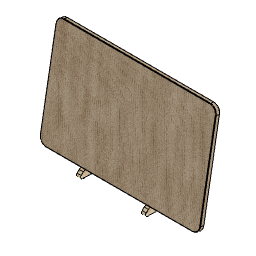
model (Autodesk Fusion 360 design; units mm, degrees)
Autodesk Fusion 360 part; units mm, degrees
note: some values were not read from the file. Chosen so that the rebuilt part matches the saved one: which bodies a step acts on; which face or edge a step refers to.
sketch "Sketch1" plane through (0, 0, 0) normal (0, 0, 1) x (1, 0, 0) in component "stock"
  line L0 (0, 0) -> (184.15, 0)
  line L1 (184.15, 0) -> (184.15, 1168.4)
  line L2 (184.15, 1168.4) -> (0, 1168.4)
  line L3 (0, 1168.4) -> (0, 0)
  line L4 (-207.15, 0) -> (-23, 0)
  line L5 (-23, 0) -> (-23, 28)
  line L6 (-23, 28) -> (-207.15, 28)
  line L7 (-207.15, 28) -> (-207.15, 0)
  line L8 (-207.15, 30) -> (-23, 30)
  line L9 (-23, 30) -> (-23, 58)
  line L10 (-207.15, 58) -> (-207.15, 30)
  line L11 (-23, 58) -> (-207.15, 58)
  line L12 (-207.15, 60) -> (-23, 60)
  line L13 (-23, 60) -> (-23, 88)
  line L14 (-207.15, 88) -> (-207.15, 60)
  line L15 (-23, 88) -> (-207.15, 88)
  line L16 (-207.15, 90) -> (-23, 90)
  line L17 (-23, 90) -> (-23, 118)
  line L18 (-207.15, 118) -> (-207.15, 90)
  line L19 (-23, 118) -> (-207.15, 118)
  line L20 (-207.15, 120) -> (-23, 120)
  line L21 (-23, 120) -> (-23, 148)
  line L22 (-207.15, 148) -> (-207.15, 120)
  line L23 (-23, 148) -> (-207.15, 148)
  line L24 (-207.15, 150) -> (-23, 150)
  line L25 (-23, 150) -> (-23, 178)
  line L26 (-207.15, 178) -> (-207.15, 150)
  line L27 (-23, 178) -> (-207.15, 178)
  line L28 (-207.15, 180) -> (-23, 180)
  line L29 (-23, 180) -> (-23, 208)
  line L30 (-207.15, 208) -> (-207.15, 180)
  line L31 (-23, 208) -> (-207.15, 208)
  line L32 (-207.15, 210) -> (-23, 210)
  line L33 (-23, 210) -> (-23, 238)
  line L34 (-207.15, 238) -> (-207.15, 210)
  line L35 (-23, 238) -> (-207.15, 238)
  line L36 (-207.15, 240) -> (-23, 240)
  line L37 (-23, 240) -> (-23, 268)
  line L38 (-207.15, 268) -> (-207.15, 240)
  line L39 (-23, 268) -> (-207.15, 268)
  line L40 (-207.15, 270) -> (-23, 270)
  line L41 (-23, 270) -> (-23, 298)
  line L42 (-207.15, 298) -> (-207.15, 270)
  line L43 (-23, 298) -> (-207.15, 298)
  line L44 (-207.15, 300) -> (-23, 300)
  line L45 (-23, 300) -> (-23, 328)
  line L46 (-207.15, 328) -> (-207.15, 300)
  line L47 (-23, 328) -> (-207.15, 328)
  line L48 (-207.15, 330) -> (-23, 330)
  line L49 (-23, 330) -> (-23, 358)
  line L50 (-207.15, 358) -> (-207.15, 330)
  line L51 (-23, 358) -> (-207.15, 358)
  line L52 (-207.15, 360) -> (-23, 360)
  line L53 (-23, 360) -> (-23, 388)
  line L54 (-207.15, 388) -> (-207.15, 360)
  line L55 (-23, 388) -> (-207.15, 388)
  line L56 (-207.15, 390) -> (-23, 390)
  line L57 (-23, 390) -> (-23, 418)
  line L58 (-207.15, 418) -> (-207.15, 390)
  line L59 (-23, 418) -> (-207.15, 418)
  line L60 (-207.15, 420) -> (-23, 420)
  line L61 (-23, 420) -> (-23, 448)
  line L62 (-207.15, 448) -> (-207.15, 420)
  line L63 (-23, 448) -> (-207.15, 448)
  line L64 (-207.15, 450) -> (-23, 450)
  line L65 (-23, 450) -> (-23, 478)
  line L66 (-207.15, 478) -> (-207.15, 450)
  line L67 (-23, 478) -> (-207.15, 478)
  line L68 (-207.15, 480) -> (-23, 480)
  line L69 (-23, 480) -> (-23, 508)
  line L70 (-207.15, 508) -> (-207.15, 480)
  line L71 (-23, 508) -> (-207.15, 508)
  line L72 (-207.15, 510) -> (-23, 510)
  line L73 (-23, 510) -> (-23, 538)
  line L74 (-207.15, 538) -> (-207.15, 510)
  line L75 (-23, 538) -> (-207.15, 538)
  line L76 (-207.15, 540) -> (-23, 540)
  line L77 (-23, 540) -> (-23, 568)
  line L78 (-207.15, 568) -> (-207.15, 540)
  line L79 (-23, 568) -> (-207.15, 568)
  line L80 (-207.15, 570) -> (-23, 570)
  line L81 (-23, 570) -> (-23, 598)
  line L82 (-207.15, 598) -> (-207.15, 570)
  line L83 (-23, 598) -> (-207.15, 598)
  line L84 (-207.15, 600) -> (-23, 600)
  line L85 (-23, 600) -> (-23, 628)
  line L86 (-207.15, 628) -> (-207.15, 600)
  line L87 (-23, 628) -> (-207.15, 628)
  line L88 (-207.15, 630) -> (-23, 630)
  line L89 (-23, 630) -> (-23, 658)
  line L90 (-207.15, 658) -> (-207.15, 630)
  line L91 (-23, 658) -> (-207.15, 658)
  line L92 (-207.15, 660) -> (-23, 660)
  line L93 (-23, 660) -> (-23, 688)
  line L94 (-207.15, 688) -> (-207.15, 660)
  line L95 (-23, 688) -> (-207.15, 688)
  line L96 (-207.15, 690) -> (-23, 690)
  line L97 (-23, 690) -> (-23, 718)
  line L98 (-207.15, 718) -> (-207.15, 690)
  line L99 (-23, 718) -> (-207.15, 718)
  line L100 (-207.15, 720) -> (-23, 720)
  line L101 (-23, 720) -> (-23, 748)
  line L102 (-207.15, 748) -> (-207.15, 720)
  line L103 (-23, 748) -> (-207.15, 748)
  line L104 (-207.15, 750) -> (-23, 750)
  line L105 (-23, 750) -> (-23, 778)
  line L106 (-207.15, 778) -> (-207.15, 750)
  line L107 (-23, 778) -> (-207.15, 778)
  line L108 (-207.15, 780) -> (-23, 780)
  line L109 (-23, 780) -> (-23, 808)
  line L110 (-207.15, 808) -> (-207.15, 780)
  line L111 (-23, 808) -> (-207.15, 808)
  line L112 (-207.15, 810) -> (-23, 810)
  line L113 (-23, 810) -> (-23, 838)
  line L114 (-207.15, 838) -> (-207.15, 810)
  line L115 (-23, 838) -> (-207.15, 838)
  line L116 (-207.15, 840) -> (-23, 840)
  line L117 (-23, 840) -> (-23, 868)
  line L118 (-207.15, 868) -> (-207.15, 840)
  line L119 (-23, 868) -> (-207.15, 868)
  line L120 (-207.15, 870) -> (-23, 870)
  line L121 (-23, 870) -> (-23, 898)
  line L122 (-207.15, 898) -> (-207.15, 870)
  line L123 (-23, 898) -> (-207.15, 898)
  line L124 (-207.15, 900) -> (-23, 900)
  line L125 (-23, 900) -> (-23, 928)
  line L126 (-207.15, 928) -> (-207.15, 900)
  line L127 (-23, 928) -> (-207.15, 928)
  line L128 (-207.15, 930) -> (-23, 930)
  line L129 (-23, 930) -> (-23, 958)
  line L130 (-207.15, 958) -> (-207.15, 930)
  line L131 (-23, 958) -> (-207.15, 958)
  line L132 (-207.15, 960) -> (-23, 960)
  line L133 (-23, 960) -> (-23, 988)
  line L134 (-207.15, 988) -> (-207.15, 960)
  line L135 (-23, 988) -> (-207.15, 988)
  line L136 (207.15, 1168.4) -> (207.15, 0)
  line L137 (207.15, 0) -> (391.3, 0)
  line L138 (391.3, 1168.4) -> (207.15, 1168.4)
  line L139 (391.3, 0) -> (391.3, 1168.4)
  line L140 (414.3, 1168.4) -> (414.3, 0)
  line L141 (414.3, 0) -> (598.45, 0)
  line L142 (598.45, 1168.4) -> (414.3, 1168.4)
  line L143 (598.45, 0) -> (598.45, 1168.4)
  line L144 (-207.15, 990) -> (-23, 990)
  line L145 (-23, 990) -> (-23, 1018)
  line L146 (-207.15, 1018) -> (-207.15, 990)
  line L147 (-23, 1018) -> (-207.15, 1018)
  dimension "d4" = 184.15
  dimension "d5" = 1168.4
  dimension "d19" = 184.15
  dimension "d20" = 28
  dimension "d25" = 0
  dimension "d26" = 30
  dimension "d27" = 23
  dimension "d30" = 207.15
  dimension "d31" = 0
  constraint horizontal L0
  constraint vertical L1
  constraint horizontal L2
  constraint vertical L3
  constraint coincident L0.start L3.end
  constraint horizontal L4
  constraint vertical L5
  constraint horizontal L6
  constraint vertical L7
  constraint collinear L0 L4
  measures "d4" distance of L1.end L2.end
  measures "d5" distance of L0.start L2.end
  measures "d19" distance of L4.start L4.end
  measures "d20" distance of L4.start L6.end
  measures "d27" distance of L3 L5
sketch "Sketch1 (2)" plane through (0, 0, 0) normal (0, 0, 1) x (1, 0, 0) in component "layout"
  line L0 (-795, -650) -> (-100, -650)
  line L1 (-100, -650) -> (-100, -200)
  line L2 (-100, -200) -> (-795, -200)
  line L3 (-795, -200) -> (-795, -650)
  line L4 (100, -200) -> (146.5, -200)
  line L5 (146.5, -200) -> (146.5, -384.15)
  line L6 (146.5, -384.15) -> (100, -384.15)
  line L7 (100, -384.15) -> (100, -200)
  line L8 (100, -200) -> (795, -200) construction
  line L9 (795, -200) -> (795, -650) construction
  line L10 (795, -650) -> (100, -650) construction
  line L11 (100, -650) -> (100, -200) construction
  line L12 (193, -384.15) -> (193, -200)
  line L13 (193, -200) -> (239.5, -200)
  line L14 (239.5, -384.15) -> (193, -384.15)
  line L15 (239.5, -200) -> (239.5, -384.15)
  line L16 (286, -384.15) -> (286, -200)
  line L17 (286, -200) -> (332.5, -200)
  line L18 (332.5, -384.15) -> (286, -384.15)
  line L19 (332.5, -200) -> (332.5, -384.15)
  line L20 (379, -384.15) -> (379, -200)
  line L21 (379, -200) -> (425.5, -200)
  line L22 (425.5, -384.15) -> (379, -384.15)
  line L23 (425.5, -200) -> (425.5, -384.15)
  line L24 (100, -568.3) -> (100, -384.15)
  line L25 (100, -384.15) -> (146.5, -384.15)
  line L26 (146.5, -568.3) -> (100, -568.3)
  line L27 (146.5, -384.15) -> (146.5, -568.3)
  line L28 (193, -568.3) -> (193, -384.15)
  line L29 (193, -384.15) -> (239.5, -384.15)
  line L30 (239.5, -568.3) -> (193, -568.3)
  line L31 (239.5, -384.15) -> (239.5, -568.3)
  line L32 (286, -568.3) -> (286, -384.15)
  line L33 (286, -384.15) -> (332.5, -384.15)
  line L34 (332.5, -568.3) -> (286, -568.3)
  line L35 (332.5, -384.15) -> (332.5, -568.3)
  line L36 (379, -568.3) -> (379, -384.15)
  line L37 (379, -384.15) -> (425.5, -384.15)
  line L38 (425.5, -568.3) -> (379, -568.3)
  line L39 (425.5, -384.15) -> (425.5, -568.3)
  line L40 (100, -752.45) -> (100, -568.3)
  line L41 (100, -568.3) -> (146.5, -568.3)
  line L42 (146.5, -752.45) -> (100, -752.45)
  line L43 (146.5, -568.3) -> (146.5, -752.45)
  line L44 (193, -752.45) -> (193, -568.3)
  line L45 (193, -568.3) -> (239.5, -568.3)
  line L46 (239.5, -752.45) -> (193, -752.45)
  line L47 (239.5, -568.3) -> (239.5, -752.45)
  line L48 (286, -752.45) -> (286, -568.3)
  line L49 (286, -568.3) -> (332.5, -568.3)
  line L50 (332.5, -752.45) -> (286, -752.45)
  line L51 (332.5, -568.3) -> (332.5, -752.45)
  line L52 (379, -752.45) -> (379, -568.3)
  line L53 (379, -568.3) -> (425.5, -568.3)
  line L54 (425.5, -752.45) -> (379, -752.45)
  line L55 (425.5, -568.3) -> (425.5, -752.45)
  line L56 (-744.2, -599.2) -> (-150.8, -599.2) construction
  line L57 (-150.8, -599.2) -> (-150.8, -250.8) construction
  line L58 (-150.8, -250.8) -> (-744.2, -250.8) construction
  line L59 (-744.2, -250.8) -> (-744.2, -599.2) construction
  circle A0 centre (-744.2, -250.8) radius 9.525
  circle A1 centre (-150.8, -250.8) radius 9.525
  circle A2 centre (-150.8, -599.2) radius 9.525
  circle A3 centre (-744.2, -599.2) radius 9.525
  line L60 (472, -384.15) -> (472, -200)
  line L61 (472, -200) -> (518.5, -200)
  line L62 (518.5, -384.15) -> (472, -384.15)
  line L63 (518.5, -200) -> (518.5, -384.15)
  line L64 (565, -384.15) -> (565, -200)
  line L65 (565, -200) -> (611.5, -200)
  line L66 (611.5, -384.15) -> (565, -384.15)
  line L67 (611.5, -200) -> (611.5, -384.15)
  line L68 (658, -384.15) -> (658, -200)
  line L69 (658, -200) -> (704.5, -200)
  line L70 (704.5, -384.15) -> (658, -384.15)
  line L71 (704.5, -200) -> (704.5, -384.15)
  line L72 (751, -384.15) -> (751, -200)
  line L73 (751, -200) -> (797.5, -200)
  line L74 (797.5, -384.15) -> (751, -384.15)
  line L75 (797.5, -200) -> (797.5, -384.15)
  line L76 (472, -568.3) -> (472, -384.15)
  line L77 (472, -384.15) -> (518.5, -384.15)
  line L78 (518.5, -568.3) -> (472, -568.3)
  line L79 (518.5, -384.15) -> (518.5, -568.3)
  line L80 (565, -568.3) -> (565, -384.15)
  line L81 (565, -384.15) -> (611.5, -384.15)
  line L82 (611.5, -568.3) -> (565, -568.3)
  line L83 (611.5, -384.15) -> (611.5, -568.3)
  line L84 (658, -568.3) -> (658, -384.15)
  line L85 (658, -384.15) -> (704.5, -384.15)
  line L86 (704.5, -568.3) -> (658, -568.3)
  line L87 (704.5, -384.15) -> (704.5, -568.3)
  line L88 (751, -568.3) -> (751, -384.15)
  line L89 (751, -384.15) -> (797.5, -384.15)
  line L90 (797.5, -568.3) -> (751, -568.3)
  line L91 (797.5, -384.15) -> (797.5, -568.3)
  line L92 (472, -752.45) -> (472, -568.3)
  line L93 (472, -568.3) -> (518.5, -568.3)
  line L94 (518.5, -752.45) -> (472, -752.45)
  line L95 (518.5, -568.3) -> (518.5, -752.45)
  line L96 (565, -752.45) -> (565, -568.3)
  line L97 (565, -568.3) -> (611.5, -568.3)
  line L98 (611.5, -752.45) -> (565, -752.45)
  line L99 (611.5, -568.3) -> (611.5, -752.45)
  line L100 (658, -752.45) -> (658, -568.3)
  line L101 (658, -568.3) -> (704.5, -568.3)
  line L102 (704.5, -752.45) -> (658, -752.45)
  line L103 (704.5, -568.3) -> (704.5, -752.45)
  line L104 (751, -752.45) -> (751, -568.3)
  line L105 (751, -568.3) -> (797.5, -568.3)
  line L106 (797.5, -752.45) -> (751, -752.45)
  line L107 (797.5, -568.3) -> (797.5, -752.45)
  line L108 (146.5, -292.075) -> (193, -292.075)
  line L109 (193, -292.075) -> (193, -107.925)
  line L110 (193, -107.925) -> (146.5, -107.925)
  line L111 (146.5, -107.925) -> (146.5, -292.075)
  line L112 (286, -292.075) -> (286, -107.925)
  line L113 (286, -107.925) -> (239.5, -107.925)
  line L114 (239.5, -107.925) -> (239.5, -292.075)
  line L115 (239.5, -292.075) -> (286, -292.075)
  line L116 (379, -292.075) -> (379, -107.925)
  line L117 (379, -107.925) -> (332.5, -107.925)
  line L118 (332.5, -107.925) -> (332.5, -292.075)
  line L119 (332.5, -292.075) -> (379, -292.075)
  line L120 (472, -292.075) -> (472, -107.925)
  line L121 (472, -107.925) -> (425.5, -107.925)
  line L122 (425.5, -107.925) -> (425.5, -292.075)
  line L123 (425.5, -292.075) -> (472, -292.075)
  line L124 (565, -292.075) -> (565, -107.925)
  line L125 (565, -107.925) -> (518.5, -107.925)
  line L126 (518.5, -107.925) -> (518.5, -292.075)
  line L127 (518.5, -292.075) -> (565, -292.075)
  line L128 (658, -292.075) -> (658, -107.925)
  line L129 (658, -107.925) -> (611.5, -107.925)
  line L130 (611.5, -107.925) -> (611.5, -292.075)
  line L131 (611.5, -292.075) -> (658, -292.075)
  line L132 (751, -292.075) -> (751, -107.925)
  line L133 (751, -107.925) -> (704.5, -107.925)
  line L134 (704.5, -107.925) -> (704.5, -292.075)
  line L135 (704.5, -292.075) -> (751, -292.075)
  line L136 (193, -476.225) -> (193, -292.075)
  line L137 (193, -292.075) -> (146.5, -292.075)
  line L138 (146.5, -292.075) -> (146.5, -476.225)
  line L139 (146.5, -476.225) -> (193, -476.225)
  line L140 (286, -476.225) -> (286, -292.075)
  line L141 (286, -292.075) -> (239.5, -292.075)
  line L142 (239.5, -292.075) -> (239.5, -476.225)
  line L143 (239.5, -476.225) -> (286, -476.225)
  line L144 (379, -476.225) -> (379, -292.075)
  line L145 (379, -292.075) -> (332.5, -292.075)
  line L146 (332.5, -292.075) -> (332.5, -476.225)
  line L147 (332.5, -476.225) -> (379, -476.225)
  line L148 (472, -476.225) -> (472, -292.075)
  line L149 (472, -292.075) -> (425.5, -292.075)
  line L150 (425.5, -292.075) -> (425.5, -476.225)
  line L151 (425.5, -476.225) -> (472, -476.225)
  line L152 (565, -476.225) -> (565, -292.075)
  line L153 (565, -292.075) -> (518.5, -292.075)
  line L154 (518.5, -292.075) -> (518.5, -476.225)
  line L155 (518.5, -476.225) -> (565, -476.225)
  line L156 (658, -476.225) -> (658, -292.075)
  line L157 (658, -292.075) -> (611.5, -292.075)
  line L158 (611.5, -292.075) -> (611.5, -476.225)
  line L159 (611.5, -476.225) -> (658, -476.225)
  line L160 (751, -476.225) -> (751, -292.075)
  line L161 (751, -292.075) -> (704.5, -292.075)
  line L162 (704.5, -292.075) -> (704.5, -476.225)
  line L163 (704.5, -476.225) -> (751, -476.225)
  line L164 (193, -660.375) -> (193, -476.225)
  line L165 (193, -476.225) -> (146.5, -476.225)
  line L166 (146.5, -476.225) -> (146.5, -660.375)
  line L167 (146.5, -660.375) -> (193, -660.375)
  line L168 (286, -660.375) -> (286, -476.225)
  line L169 (286, -476.225) -> (239.5, -476.225)
  line L170 (239.5, -476.225) -> (239.5, -660.375)
  line L171 (239.5, -660.375) -> (286, -660.375)
  line L172 (379, -660.375) -> (379, -476.225)
  line L173 (379, -476.225) -> (332.5, -476.225)
  line L174 (332.5, -476.225) -> (332.5, -660.375)
  line L175 (332.5, -660.375) -> (379, -660.375)
  line L176 (472, -660.375) -> (472, -476.225)
  line L177 (472, -476.225) -> (425.5, -476.225)
  line L178 (425.5, -476.225) -> (425.5, -660.375)
  line L179 (425.5, -660.375) -> (472, -660.375)
  line L180 (565, -660.375) -> (565, -476.225)
  line L181 (565, -476.225) -> (518.5, -476.225)
  line L182 (518.5, -476.225) -> (518.5, -660.375)
  line L183 (518.5, -660.375) -> (565, -660.375)
  line L184 (658, -660.375) -> (658, -476.225)
  line L185 (658, -476.225) -> (611.5, -476.225)
  line L186 (611.5, -476.225) -> (611.5, -660.375)
  line L187 (611.5, -660.375) -> (658, -660.375)
  line L188 (751, -660.375) -> (751, -476.225)
  line L189 (751, -476.225) -> (704.5, -476.225)
  line L190 (704.5, -476.225) -> (704.5, -660.375)
  line L191 (704.5, -660.375) -> (751, -660.375)
  dimension "d14" = 695
  dimension "d15" = 450
  dimension "d36" = 200
  dimension "d38" = 100
  dimension "d39" = 46.5
  dimension "d40" = 184.15
  dimension "d41" = 200
  dimension "d42" = 695
  dimension "d43" = 450
  dimension "d46" = 93
  dimension "d79" = 19.05
  dimension "d80" = 19.05
  dimension "d81" = 19.05
  dimension "d82" = 19.05
  dimension "d98" = 93
  constraint horizontal L0
  constraint vertical L1
  constraint horizontal L2
  constraint vertical L3
  constraint horizontal L4
  constraint vertical L5
  constraint horizontal L6
  constraint vertical L7
  constraint collinear L2 L4
  constraint horizontal L8
  constraint vertical L9
  constraint horizontal L10
  constraint vertical L11
  constraint coincident L58.end L59.start
  constraint coincident L57.end L58.start
  constraint coincident L56.end L57.start
  constraint coincident L56.start L59.end
  constraint horizontal L108
  constraint vertical L109
  constraint horizontal L110
  constraint vertical L111
  constraint midpoint L5 L108.start
  constraint collinear L12 L109
  constraint equal L7 L111
  measures "d14" distance of L1.end L2.end
  measures "d15" distance of L0.start L2.end
  measures "d36" distance of L2 origin
  measures "d38" distance of origin L1
  measures "d39" distance of L4.start L4.end
  measures "d40" distance of L4.start L6.end
  measures "d41" distance of L1 L7
  measures "d42" distance of L4.start L8.end
  measures "d43" distance of L8.end L9.end
  measures "d79" diameter of A0
  measures "d80" diameter of A1
  measures "d81" diameter of A3
  measures "d82" diameter of A2
extrude "Extrude2" add sketch "Sketch1" along normal blind 46.5 contours L0 L1 L2 L3 makes body 1 in component "stock"
extrude "Extrude3" add sketch "Sketch1" along normal blind 46.5 separate body contours L4 L5 L6 L7 makes body 2 in component "stock"
sketch "Sketch2" plane through (0, 0, 0) normal (0, 0, 1) x (1, 0, 0) in component "brick (outdated)"
  line L0 (0, -0.2486) -> (129.54, -0.2486)
  line L1 (129.54, -0.2486) -> (129.54, 46.2514)
  line L2 (129.54, 46.2514) -> (0, 46.2514)
  line L3 (0, 46.2514) -> (0, -0.2486)
  line L4 (129.54, -0.2486) -> (302.26, -0.2486)
  line L5 (302.26, -0.2486) -> (302.26, 46.2514)
  line L6 (302.26, 46.2514) -> (129.54, 46.2514)
  line L7 (129.54, 46.2514) -> (129.54, -0.2486)
  line L8 (302.26, -0.2486) -> (431.8, -0.2486)
  line L9 (431.8, -0.2486) -> (431.8, 46.2514)
  line L10 (431.8, 46.2514) -> (302.26, 46.2514)
  line L11 (302.26, 46.2514) -> (302.26, -0.2486)
  line L12 (431.8, -0.2486) -> (584.2, -0.2486)
  line L13 (584.2, -0.2486) -> (584.2, 46.2514)
  line L14 (584.2, 46.2514) -> (431.8, 46.2514)
  line L15 (431.8, 46.2514) -> (431.8, -0.2486)
  line L16 (584.2, -0.2486) -> (736.6, -0.2486)
  line L17 (736.6, -0.2486) -> (736.6, 46.2514)
  line L18 (736.6, 46.2514) -> (584.2, 46.2514)
  line L19 (584.2, 46.2514) -> (584.2, -0.2486)
  line L20 (736.6, -0.2486) -> (909.32, -0.2486)
  line L21 (909.32, -0.2486) -> (909.32, 46.2514)
  line L22 (909.32, 46.2514) -> (736.6, 46.2514)
  line L23 (736.6, 46.2514) -> (736.6, -0.2486)
  line L24 (606.8221, -46.2418) -> (779.5421, -46.3005)
  line L25 (324.88, 0.0519) -> (172.4798, 0.0264)
  line L26 (606.821, -46.2418) -> (606.8213, 0.101)
  line L27 (477.2805, 0.0783) -> (477.281, -46.1978)
  line L28 (324.88, 0.0519) -> (324.8803, -46.146)
  line L29 (324.8803, -46.146) -> (477.2803, -46.1978)
  line L30 (172.4798, 0.0264) -> (-0.2403, 0)
  line L31 (477.2805, 0.0783) -> (324.88, 0.0519)
  line L32 (-0.2403, 0) -> (-0.2404, -46.0356)
  line L33 (-0.2404, -46.0356) -> (172.4796, -46.0942)
  line L34 (172.4796, -46.0942) -> (172.4798, 0.0264)
  line L35 (172.4798, 0.0264) -> (172.4798, -46.0942)
  line L36 (324.8798, -46.146) -> (324.88, 0.0519)
  line L37 (779.5437, -46.3005) -> (909.0837, -46.3445)
  line L38 (779.5421, -46.3005) -> (779.5425, 0.1322)
  line L39 (477.281, -46.1978) -> (606.821, -46.2418)
  line L40 (909.078, 0.1555) -> (779.5425, 0.1322)
  line L41 (909.0837, -46.3445) -> (909.078, 0.1555)
  line L42 (606.8213, 0.101) -> (477.2805, 0.0783)
  line L43 (779.5425, 0.1322) -> (606.8213, 0.101)
  line L44 (779.5425, 0.1322) -> (779.5437, -46.3005)
  line L45 (606.8213, 0.101) -> (606.8221, -46.2418)
  line L46 (172.4798, -46.0942) -> (324.8798, -46.146)
  line L47 (477.2803, -46.1978) -> (477.2805, 0.0783)
  line L48 (-0.2404, -139.0356) -> (172.4796, -139.0942)
  line L49 (324.88, -92.9481) -> (324.8803, -139.146)
  line L50 (129.54, -46.7486) -> (0, -46.7486)
  line L51 (584.2, -93.2486) -> (736.6, -93.2486)
  line L52 (431.8, -93.2486) -> (584.2, -93.2486)
  line L53 (324.88, -92.9481) -> (172.4798, -92.9736)
  line L54 (477.281, -139.1978) -> (606.821, -139.2418)
  line L55 (584.2, -46.7486) -> (584.2, -93.2486)
  line L56 (606.8213, -92.899) -> (477.2805, -92.9217)
  line L57 (584.2, -93.2486) -> (584.2, -46.7486)
  line L58 (324.8798, -139.146) -> (324.88, -92.9481)
  line L59 (172.4798, -92.9736) -> (172.4798, -139.0942)
  line L60 (302.26, -93.2486) -> (302.26, -46.7486)
  line L61 (736.6, -46.7486) -> (584.2, -46.7486)
  line L62 (736.6, -93.2486) -> (909.32, -93.2486)
  line L63 (606.8213, -92.899) -> (606.8221, -139.2418)
  line L64 (736.6, -93.2486) -> (736.6, -46.7486)
  line L65 (909.32, -93.2486) -> (909.32, -46.7486)
  line L66 (909.0837, -139.3445) -> (909.078, -92.8445)
  line L67 (909.32, -46.7486) -> (736.6, -46.7486)
  line L68 (736.6, -46.7486) -> (736.6, -93.2486)
  line L69 (606.821, -139.2418) -> (606.8213, -92.899)
  line L70 (779.5437, -139.3005) -> (909.0837, -139.3445)
  line L71 (779.5425, -92.8678) -> (606.8213, -92.899)
  line L72 (779.5421, -139.3005) -> (779.5425, -92.8678)
  line L73 (909.078, -92.8445) -> (779.5425, -92.8678)
  line L74 (779.5425, -92.8678) -> (779.5437, -139.3005)
  line L75 (606.8221, -139.2418) -> (779.5421, -139.3005)
  line L76 (172.4798, -139.0942) -> (324.8798, -139.146)
  line L77 (129.54, -93.2486) -> (302.26, -93.2486)
  line L78 (477.2803, -139.1978) -> (477.2805, -92.9217)
  line L79 (302.26, -46.7486) -> (129.54, -46.7486)
  line L80 (172.4798, -92.9736) -> (-0.2403, -93)
  line L81 (431.8, -93.2486) -> (431.8, -46.7486)
  line L82 (477.2805, -92.9217) -> (324.88, -92.9481)
  line L83 (431.8, -46.7486) -> (302.26, -46.7486)
  line L84 (477.2805, -92.9217) -> (477.281, -139.1978)
  line L85 (129.54, -93.2486) -> (129.54, -46.7486)
  line L86 (0, -93.2486) -> (129.54, -93.2486)
  line L87 (0, -46.7486) -> (0, -93.2486)
  line L88 (302.26, -46.7486) -> (302.26, -93.2486)
  line L89 (584.2, -46.7486) -> (431.8, -46.7486)
  line L90 (172.4796, -139.0942) -> (172.4798, -92.9736)
  line L91 (129.54, -46.7486) -> (129.54, -93.2486)
  line L92 (431.8, -46.7486) -> (431.8, -93.2486)
  line L93 (-0.2403, -93) -> (-0.2404, -139.0356)
  line L94 (302.26, -93.2486) -> (431.8, -93.2486)
  line L95 (324.8803, -139.146) -> (477.2803, -139.1978)
  line L96 (-0.2404, -232.0356) -> (172.4796, -232.0942)
  line L97 (324.88, -185.9481) -> (324.8803, -232.146)
  line L98 (129.54, -139.7486) -> (0, -139.7486)
  line L99 (584.2, -186.2486) -> (736.6, -186.2486)
  line L100 (431.8, -186.2486) -> (584.2, -186.2486)
  line L101 (324.88, -185.9481) -> (172.4798, -185.9736)
  line L102 (477.281, -232.1978) -> (606.821, -232.2418)
  line L103 (584.2, -139.7486) -> (584.2, -186.2486)
  line L104 (606.8213, -185.899) -> (477.2805, -185.9217)
  line L105 (584.2, -186.2486) -> (584.2, -139.7486)
  line L106 (324.8798, -232.146) -> (324.88, -185.9481)
  line L107 (172.4798, -185.9736) -> (172.4798, -232.0942)
  line L108 (302.26, -186.2486) -> (302.26, -139.7486)
  line L109 (736.6, -139.7486) -> (584.2, -139.7486)
  line L110 (736.6, -186.2486) -> (909.32, -186.2486)
  line L111 (606.8213, -185.899) -> (606.8221, -232.2418)
  line L112 (736.6, -186.2486) -> (736.6, -139.7486)
  line L113 (909.32, -186.2486) -> (909.32, -139.7486)
  line L114 (909.0837, -232.3445) -> (909.078, -185.8445)
  line L115 (909.32, -139.7486) -> (736.6, -139.7486)
  line L116 (736.6, -139.7486) -> (736.6, -186.2486)
  line L117 (606.821, -232.2418) -> (606.8213, -185.899)
  line L118 (779.5437, -232.3005) -> (909.0837, -232.3445)
  line L119 (779.5425, -185.8678) -> (606.8213, -185.899)
  line L120 (779.5421, -232.3005) -> (779.5425, -185.8678)
  line L121 (909.078, -185.8445) -> (779.5425, -185.8678)
  line L122 (779.5425, -185.8678) -> (779.5437, -232.3005)
  line L123 (606.8221, -232.2418) -> (779.5421, -232.3005)
  line L124 (172.4798, -232.0942) -> (324.8798, -232.146)
  line L125 (129.54, -186.2486) -> (302.26, -186.2486)
  line L126 (477.2803, -232.1978) -> (477.2805, -185.9217)
  line L127 (302.26, -139.7486) -> (129.54, -139.7486)
  line L128 (172.4798, -185.9736) -> (-0.2403, -186)
  line L129 (431.8, -186.2486) -> (431.8, -139.7486)
  line L130 (477.2805, -185.9217) -> (324.88, -185.9481)
  line L131 (431.8, -139.7486) -> (302.26, -139.7486)
  line L132 (477.2805, -185.9217) -> (477.281, -232.1978)
  line L133 (129.54, -186.2486) -> (129.54, -139.7486)
  line L134 (0, -186.2486) -> (129.54, -186.2486)
  line L135 (0, -139.7486) -> (0, -186.2486)
  line L136 (302.26, -139.7486) -> (302.26, -186.2486)
  line L137 (584.2, -139.7486) -> (431.8, -139.7486)
  line L138 (172.4796, -232.0942) -> (172.4798, -185.9736)
  line L139 (129.54, -139.7486) -> (129.54, -186.2486)
  line L140 (431.8, -139.7486) -> (431.8, -186.2486)
  line L141 (-0.2403, -186) -> (-0.2404, -232.0356)
  line L142 (302.26, -186.2486) -> (431.8, -186.2486)
  line L143 (324.8803, -232.146) -> (477.2803, -232.1978)
  line L144 (-0.2404, -325.0356) -> (172.4796, -325.0942)
  line L145 (324.88, -278.9481) -> (324.8803, -325.146)
  line L146 (129.54, -232.7486) -> (0, -232.7486)
  line L147 (584.2, -279.2486) -> (736.6, -279.2486)
  line L148 (431.8, -279.2486) -> (584.2, -279.2486)
  line L149 (324.88, -278.9481) -> (172.4798, -278.9736)
  line L150 (477.281, -325.1978) -> (606.821, -325.2418)
  line L151 (584.2, -232.7486) -> (584.2, -279.2486)
  line L152 (606.8213, -278.899) -> (477.2805, -278.9217)
  line L153 (584.2, -279.2486) -> (584.2, -232.7486)
  line L154 (324.8798, -325.146) -> (324.88, -278.9481)
  line L155 (172.4798, -278.9736) -> (172.4798, -325.0942)
  line L156 (302.26, -279.2486) -> (302.26, -232.7486)
  line L157 (736.6, -232.7486) -> (584.2, -232.7486)
  line L158 (736.6, -279.2486) -> (909.32, -279.2486)
  line L159 (606.8213, -278.899) -> (606.8221, -325.2418)
  line L160 (736.6, -279.2486) -> (736.6, -232.7486)
  line L161 (909.32, -279.2486) -> (909.32, -232.7486)
  line L162 (909.0837, -325.3445) -> (909.078, -278.8445)
  line L163 (909.32, -232.7486) -> (736.6, -232.7486)
  line L164 (736.6, -232.7486) -> (736.6, -279.2486)
  line L165 (606.821, -325.2418) -> (606.8213, -278.899)
  line L166 (779.5437, -325.3005) -> (909.0837, -325.3445)
  line L167 (779.5425, -278.8678) -> (606.8213, -278.899)
  line L168 (779.5421, -325.3005) -> (779.5425, -278.8678)
  line L169 (909.078, -278.8445) -> (779.5425, -278.8678)
  line L170 (779.5425, -278.8678) -> (779.5437, -325.3005)
  line L171 (606.8221, -325.2418) -> (779.5421, -325.3005)
  line L172 (172.4798, -325.0942) -> (324.8798, -325.146)
  line L173 (129.54, -279.2486) -> (302.26, -279.2486)
  line L174 (477.2803, -325.1978) -> (477.2805, -278.9217)
  line L175 (302.26, -232.7486) -> (129.54, -232.7486)
  line L176 (172.4798, -278.9736) -> (-0.2403, -279)
  line L177 (431.8, -279.2486) -> (431.8, -232.7486)
  line L178 (477.2805, -278.9217) -> (324.88, -278.9481)
  line L179 (431.8, -232.7486) -> (302.26, -232.7486)
  line L180 (477.2805, -278.9217) -> (477.281, -325.1978)
  line L181 (129.54, -279.2486) -> (129.54, -232.7486)
  line L182 (0, -279.2486) -> (129.54, -279.2486)
  line L183 (0, -232.7486) -> (0, -279.2486)
  line L184 (302.26, -232.7486) -> (302.26, -279.2486)
  line L185 (584.2, -232.7486) -> (431.8, -232.7486)
  line L186 (172.4796, -325.0942) -> (172.4798, -278.9736)
  line L187 (129.54, -232.7486) -> (129.54, -279.2486)
  line L188 (431.8, -232.7486) -> (431.8, -279.2486)
  line L189 (-0.2403, -279) -> (-0.2404, -325.0356)
  line L190 (302.26, -279.2486) -> (431.8, -279.2486)
  line L191 (324.8803, -325.146) -> (477.2803, -325.1978)
  line L192 (-0.2404, -418.0356) -> (172.4796, -418.0942)
  line L193 (324.88, -371.9481) -> (324.8803, -418.146)
  line L194 (129.54, -325.7486) -> (0, -325.7486)
  line L195 (584.2, -372.2486) -> (736.6, -372.2486)
  line L196 (431.8, -372.2486) -> (584.2, -372.2486)
  line L197 (324.88, -371.9481) -> (172.4798, -371.9736)
  line L198 (477.281, -418.1978) -> (606.821, -418.2418)
  line L199 (584.2, -325.7486) -> (584.2, -372.2486)
  line L200 (606.8213, -371.899) -> (477.2805, -371.9217)
  line L201 (584.2, -372.2486) -> (584.2, -325.7486)
  line L202 (324.8798, -418.146) -> (324.88, -371.9481)
  line L203 (172.4798, -371.9736) -> (172.4798, -418.0942)
  line L204 (302.26, -372.2486) -> (302.26, -325.7486)
  line L205 (736.6, -325.7486) -> (584.2, -325.7486)
  line L206 (736.6, -372.2486) -> (909.32, -372.2486)
  line L207 (606.8213, -371.899) -> (606.8221, -418.2418)
  line L208 (736.6, -372.2486) -> (736.6, -325.7486)
  line L209 (909.32, -372.2486) -> (909.32, -325.7486)
  line L210 (909.0837, -418.3445) -> (909.078, -371.8445)
  line L211 (909.32, -325.7486) -> (736.6, -325.7486)
  line L212 (736.6, -325.7486) -> (736.6, -372.2486)
  line L213 (606.821, -418.2418) -> (606.8213, -371.899)
  line L214 (779.5437, -418.3005) -> (909.0837, -418.3445)
  line L215 (779.5425, -371.8678) -> (606.8213, -371.899)
  line L216 (779.5421, -418.3005) -> (779.5425, -371.8678)
  line L217 (909.078, -371.8445) -> (779.5425, -371.8678)
  line L218 (779.5425, -371.8678) -> (779.5437, -418.3005)
  line L219 (606.8221, -418.2418) -> (779.5421, -418.3005)
  line L220 (172.4798, -418.0942) -> (324.8798, -418.146)
  line L221 (129.54, -372.2486) -> (302.26, -372.2486)
  line L222 (477.2803, -418.1978) -> (477.2805, -371.9217)
  line L223 (302.26, -325.7486) -> (129.54, -325.7486)
  line L224 (172.4798, -371.9736) -> (-0.2403, -372)
  line L225 (431.8, -372.2486) -> (431.8, -325.7486)
  line L226 (477.2805, -371.9217) -> (324.88, -371.9481)
  line L227 (431.8, -325.7486) -> (302.26, -325.7486)
  line L228 (477.2805, -371.9217) -> (477.281, -418.1978)
  line L229 (129.54, -372.2486) -> (129.54, -325.7486)
  line L230 (0, -372.2486) -> (129.54, -372.2486)
  line L231 (0, -325.7486) -> (0, -372.2486)
  line L232 (302.26, -325.7486) -> (302.26, -372.2486)
  line L233 (584.2, -325.7486) -> (431.8, -325.7486)
  line L234 (172.4796, -418.0942) -> (172.4798, -371.9736)
  line L235 (129.54, -325.7486) -> (129.54, -372.2486)
  line L236 (431.8, -325.7486) -> (431.8, -372.2486)
  line L237 (-0.2403, -372) -> (-0.2404, -418.0356)
  line L238 (302.26, -372.2486) -> (431.8, -372.2486)
  line L239 (324.8803, -418.146) -> (477.2803, -418.1978)
  point P0 (0, -93)
  point P1 (0, -186)
  point P2 (0, -279)
  point P3 (0, -372)
  dimension "d56" = 46.5
  dimension "d57" = 129.54
  dimension "d58" = 172.72
  dimension "d59" = 129.54
  dimension "d60" = 152.4
  dimension "d61" = 152.4
  dimension "d62" = 172.72
  dimension "d63" = 46.5
  dimension "d64" = 129.54
  dimension "d65" = 172.72
  dimension "d66" = 129.54
  dimension "d67" = 152.4
  dimension "d68" = 152.4
  dimension "d69" = 172.72
  dimension "d72" = 0
  dimension "d73" = -372
  constraint horizontal L0
  constraint vertical L1
  constraint horizontal L2
  constraint vertical L3
  constraint horizontal L4
  constraint vertical L5
  constraint horizontal L6
  constraint vertical L7
  constraint horizontal L8
  constraint vertical L9
  constraint horizontal L10
  constraint vertical L11
  constraint horizontal L12
  constraint vertical L13
  constraint horizontal L14
  constraint vertical L15
  constraint horizontal L16
  constraint vertical L17
  constraint horizontal L18
  constraint vertical L19
  constraint horizontal L20
  constraint vertical L21
  constraint horizontal L22
  constraint vertical L23
  constraint collinear L2 L6
  constraint collinear L6 L10
  constraint collinear L10 L14
  constraint collinear L14 L18
  constraint collinear L18 L22
  constraint collinear L24 L37
  constraint collinear L24 L39
  constraint collinear L29 L39
  constraint collinear L29 L46
  constraint collinear L33 L46
  measures "d56" distance of L0.start L2.end
  measures "d57" distance of L1.end L2.end
  measures "d58" distance of L5.end L1.end
  measures "d59" distance of L9.end L5.end
  measures "d60" distance of L13.end L9.end
  measures "d61" distance of L17.end L13.end
  measures "d62" distance of L21.end L17.end
  measures "d63" distance of L37.end L40.start
  measures "d64" distance of L37.start L37.end
  measures "d65" distance of L24.end L24.start
  measures "d66" distance of L27.end L26.start
  measures "d67" distance of L28.end L29.end
  measures "d68" distance of L35.end L36.start
  measures "d69" distance of L33.end L32.end
extrude "Extrude1" add sketch "Sketch1 (2)" along normal blind 28 separate body contours L0 L1 L2 L3 | A0 | A1 | A2 | A3 makes body 3
extrude "Extrude2'" add sketch "Sketch1 (2)" against normal blind 5 draft -20 separate body contours A0 | A1 | A2 | A3 makes body 4 at (-159.7184, -599.2, -1.6667) makes body 5 at (-154.0583, -242.4981, -1.6667) makes body 6 at (-737.6624, -593.134, -1.6667) makes body 7 at (-744.8665, -259.6934, -1.6667)
fillet "Fillet1" radius 3 4 faces at (-155.095, -597.2572, -5) (-152.6828, -251.0329, -5) (-748.1988, -600.6468, -5) (-746.7684, -250.8, -5) on bodies 4 5 6 7
fillet "Fillet2" radius 30 4 edges at (-795, -650, 14) (-100, -650, 14) (-795, -200, 14) (-100, -200, 14) on bodies 3
chamfer "Chamfer1" distance 12 angle 45 8 edges at (-447.5, -650, 0) (-108.7868, -641.2132, 0) (-100, -425, 0) (-108.7868, -208.7868, 0) (-447.5, -200, 0) (-786.2132, -208.7868, 0) (-795, -425, 0) (-786.2132, -641.2132, 0) on bodies 3
chamfer "Chamfer2" distance 2 angle 45 8 edges at (-447.5, -650, 28) (-108.7868, -641.2132, 28) (-100, -425, 28) (-108.7868, -208.7868, 28) (-447.5, -200, 28) (-786.2132, -208.7868, 28) (-795, -425, 28) (-786.2132, -641.2132, 28) on bodies 3
sketch "sled hole" plane through (0, 0, 46.5) normal (0, 0, 1) x (-1, 0, 0)
  line L0 (0, -1168.4) -> (0, 0)
  line L1 (0, 0) -> (-184.15, 0)
  line L2 (-184.15, 0) -> (-184.15, -1168.4)
  line L3 (-184.15, -1168.4) -> (0, -1168.4)
  line L4 (732.3228, 800.8503) -> (732.1228, 800.8503)
  line L5 (699.7228, 833.2503) -> (699.7228, 1283.4503)
  line L6 (732.1228, 1315.8503) -> (732.3228, 1315.8503)
  line L7 (764.7228, 1283.4503) -> (764.7228, 833.2503)
  arc A0 (732.3228, 800.8503) -> (764.7228, 833.2503) centre (732.3228, 833.2503) ccw
  arc A1 (699.7228, 833.2503) -> (732.1228, 800.8503) centre (732.1228, 833.2503) ccw
  arc A2 (764.7228, 1283.4503) -> (732.3228, 1315.8503) centre (732.3228, 1283.4503) ccw
  arc A3 (732.1228, 1315.8503) -> (699.7228, 1283.4503) centre (732.1228, 1283.4503) ccw
  point P0 (764.7228, 800.8503)
  point P1 (699.7228, 800.8503)
  point P2 (764.7228, 1315.8503)
  dimension "d91" = 65
  dimension "d92" = 515
  dimension "d93" = 32.4
  constraint horizontal L4
  constraint vertical L5
  constraint horizontal L6
  constraint vertical L7
  constraint coincident P0 L4
  constraint coincident P0 L7
  constraint tangent L4 A0
  constraint tangent L7 A0
  constraint coincident P1 L4
  constraint coincident P1 L5
  constraint tangent L4 A1
  constraint tangent L5 A1
  constraint equal A0 A1
  constraint coincident P2 L6
  constraint coincident P2 L7
  constraint tangent L6 A2
  constraint tangent L7 A2
  constraint equal A0 A2
  constraint tangent L5 A3
  constraint tangent L6 A3
  constraint equal A0 A3
  measures "d91" distance of P0 P1
  measures "d92" distance of P0 P2
  measures "d93" radius of A0
sketch "profile" plane through (0, 0, 0) normal (1, 0, 0) x (0, 1, 0) in component "stand"
  line L0 (39.4216, 22.748) -> (117.216, 463.9419)
  line L1 (117.216, 463.9419) -> (144.7906, 459.0797)
  line L2 (144.7906, 459.0797) -> (68.7327, 27.7339)
  line L3 (54.8313, 18) -> (41.044, 20.4311)
  line L4 (117.216, 463.9419) -> (131.0033, 463.9419) construction
  line L5 (131.0033, 463.9419) -> (131.0033, 461.5108) construction
  line L6 (0, 0) -> (30.7375, 30.7375)
  line L7 (144.7906, 335.8508) -> (144.7906, 0)
  line L8 (144.7906, 0) -> (0, 0)
  line L9 (144.7906, 459.0797) -> (144.7906, 0) construction
  line L10 (39.4216, 22.748) -> (41.044, 20.4311)
  line L11 (54.8313, 18) -> (68.7327, 27.7339)
  line L12 (106.7617, 243.4068) -> (144.7906, 236.7013) construction
  line L13 (43.475, 18) -> (126.7906, 18)
  line L14 (126.7906, 18) -> (126.7906, 292.3758)
  line L15 (114.0531, 305.1133) -> (144.7906, 335.8508)
  line L16 (30.7375, 30.7375) -> (43.475, 18)
  line L17 (126.7906, 292.3758) -> (114.0531, 305.1133)
  line L18 (85.1328, 18) -> (85.1328, 0) construction
  line L19 (126.7906, 155.1879) -> (144.7906, 155.1879) construction
  line L20 (30.7375, 30.7375) -> (30.7375, 0) construction
  line L21 (43.475, 18) -> (30.7375, 18) construction
  line L22 (30.7375, 18) -> (18, 18) construction
  line L23 (114.0531, 305.1133) -> (144.7906, 305.1133) construction
  line L24 (126.7906, 292.3758) -> (126.7906, 305.1133) construction
  line L25 (126.7906, 305.1133) -> (126.7906, 317.8508) construction
  arc A0 (120.4171, 311.4773) -> (120.4219, 298.7446) centre (126.781, 305.1133) ccw construction
  dimension "d100" = 28
  dimension "d103" = 10
  dimension "d124" = 16.9706
  dimension "d125" = 135
  dimension "d126" = 450
  dimension "d127" = 2.8284
  dimension "d128" = 135
  dimension "d129" = 18
  dimension "d130" = 90
  dimension "d131" = 90
  dimension "d133" = 9
  constraint perpendicular L0 L1
  constraint perpendicular L1 L2
  constraint perpendicular L0 L3
  constraint horizontal L4
  constraint midpoint L1 L5.end
  constraint vertical L5
  constraint midpoint L2 L12.start
  constraint coincident L9 L7.start
  constraint perpendicular L2 L12
  constraint coincident L6.start L8.end
  constraint coincident L8 L7.end
  constraint parallel L7 L14
  constraint parallel L8 L13
  constraint horizontal L8
  constraint vertical L7
  constraint vertical L9
  constraint coincident L13.end L14.start
  constraint coincident L9 L12.end
  constraint coincident L7.start L15.end
  constraint midpoint L13 L18.start
  constraint coincident L8 L18.end
  constraint perpendicular L8 L18
  constraint midpoint L14 L19.start
  constraint coincident L9 L19.end
  constraint perpendicular L7 L19
  constraint equal L18 L19
  constraint coincident L8 L20.end
  constraint perpendicular L8 L20
  constraint coincident L20 L21.end
  constraint perpendicular L20 L21
  constraint coincident L6 L22.end
  constraint perpendicular L20 L22
  constraint equal L21 L22
  constraint coincident L7 L23.end
  constraint perpendicular L7 L23
  constraint coincident L23 L24.end
  constraint perpendicular L23 L24
  constraint coincident L15 L25.end
  constraint perpendicular L23 L25
  constraint equal L24 L25
  constraint equal L20 L23
  constraint tangent L2 A0
  constraint midpoint L17 A0.end
  constraint coincident L15 A0.start
  constraint tangent L17 A0
  constraint tangent L15 A0
  constraint coincident L3.start L13
  constraint coincident L3.end L16
  measures "d100" distance of L0.end L1.end
  measures "d103" angle of L1 L4
  measures "d124" distance of L3.start L2.end
  measures "d125" angle of L2 L11
  measures "d126" distance of L1 L3
  measures "d127" distance of L0.start L3.end
  measures "d128" angle of L0 L10
  measures "d129" distance of L19.start L19.end
  measures "d130" angle of L15 L17
  measures "d131" angle of L6 L16
  measures "d133" radius of A0
extrude "Extrude1'" add sketch "profile" along normal blind 18 separate body contours L2 L6 L7 L8 L13 L14 L15 L16 L17 | L2 L15 L17 makes body 8 in component "stand"
fillet "Fillet1'" radius 9 6 edges at (9, 144.7906, 335.8508) (9, 114.0531, 305.1133) (9, 126.7906, 292.3758) (9, 0, 0) (9, 30.7375, 30.7375) (9, 43.475, 18) on bodies 8 in component "stand"
sketch "corner joint" plane through (0, 144.7906, 0) normal (0, 1, 0) x (-1, 0, 0) in component "stand"
  line L0 (0, 314.1229) -> (-18, 314.1229)
  line L1 (-18, 314.1229) -> (-18, 0)
  line L2 (-18, 0) -> (0, 0)
  line L3 (0, 0) -> (0, 314.1229)
  line L4 (0, 0) -> (-18, 0)
  line L5 (-18, 0) -> (-18, 18)
  line L6 (-18, 18) -> (0, 18)
  line L7 (0, 18) -> (0, 0)
  line L8 (-9, 18) -> (-9, 0)
  constraint horizontal L4
  constraint vertical L5
  constraint horizontal L6
  constraint vertical L7
  constraint coincident L1 L5.end
  constraint coincident L2.end L3.start
  constraint midpoint L6 L8.start
  constraint midpoint L4 L8.end
  constraint equal L4 L7
split "Split1" by plane through (0, 126.7906, 18) normal (0, -1, 0) bodies 8 makes body 9 at (0, 65.2405, 6) makes body 10 at (12, 117.7931, 305.5788) in component "stand"
combine "Combine1" operation add target body 8 tool bodies 10 in component "stand"
extrude "Extrude2''" add sketch "corner joint" against normal up to surface (18 mm away) contours L1 L2 L4 L5 L6 L8 bodies 9 in component "stand"
extrude "Extrude3'" cut sketch "corner joint" against normal up to surface (18 mm away) contours L1 L2 L4 L5 L6 L8 bodies 8 in component "stand"
ref_plane "WorkPlane1" through (150, 72.3953, 167.9254) normal (-1, 0, 0) x (0, -1, 0) in component "stand"
mirror "Mirror2" about plane through (150, 72.3953, 167.9254) normal (-1, 0, 0) of bodies 8 9 makes body 11 at (300, 138.7906, 200.9236) makes body 12 at (282, 71.2405, 6) in component "stand"
sketch "stretcher" plane through (0, 126.7906, 0) normal (0, -1, 0) x (1, 0, 0) in component "stand"
  line L0 (9, 0) -> (9, 18)
  line L1 (9, 18) -> (18, 18)
  line L2 (18, 18) -> (18, 288.6479)
  line L3 (18, 288.6479) -> (0, 288.6479)
  line L4 (0, 288.6479) -> (0, 0)
  line L5 (0, 0) -> (9, 0)
  arc A0 (150, 125) -> (-15.0485, 101.8526) centre (150, -475) ccw
  line L6 (282, 18) -> (282, 288.6479)
  line L7 (18, 245) -> (150, 245) construction
  line L8 (150, 245) -> (282, 245) construction
  line L9 (150, 245) -> (150, 125) construction
  line L10 (150, 125) -> (282, 125) construction
  arc A1 (150, 143) -> (-20, 119.1582) centre (150, -475) ccw
  line L11 (-15.0485, 101.8526) -> (-20, 119.1582)
  line L12 (-15.0485, 101.8526) -> (-64.2191, 87.784) construction
  line L13 (150, 143) -> (150, 125)
  dimension "d167" = 18
  dimension "d169" = 125
  dimension "d170" = 20
  dimension "d171" = 600
  constraint coincident L2 L7.start
  constraint perpendicular L2 L7
  constraint coincident L6 L8.end
  constraint perpendicular L6 L8
  constraint equal L7 L8
  constraint perpendicular L8 L9
  constraint tangent A0 L10
  constraint perpendicular L9 L10
  constraint coincident L9 A1.start
  constraint coincident A0.centre A1.centre
  constraint coincident L6 L10.end
  constraint tangent A0 L12
  constraint perpendicular L11 L12
  measures "d167" distance of A0.start A1.start
  measures "d169" vertical distance of L4.end A0.start
  measures "d170" distance of L4 A1.end
  measures "d171" radius of A0
extrude "Extrude8" add sketch "stretcher" along normal blind 5 separate body contours L4 A0 A1 L11 | L2 L4 A0 A1 | L2 A0 A1 L13 makes body 13 in component "stand"
extrude "Extrude9" add sketch "stretcher" against normal blind 13 contours L4 A0 A1 L11 | L2 A0 A1 L13 bodies 13 in component "stand"
extrude "Extrude10" add sketch "stretcher" against normal blind 6.5 contours L2 L4 A0 A1 bodies 13 in component "stand"
mirror "Mirror3" about plane through (150, 72.3953, 167.9254) normal (-1, 0, 0) of bodies 13 merged in component "stand"
combine "Combine2" operation cut target body 8 tool bodies 13 keep tools in component "stand"
combine "Combine3" operation cut target body 11 tool bodies 13 keep tools in component "stand"
move_body "Move1" bodies 6 5 4 3 7 to x (1, 0, 0) y (0, 0.173648, 0.984808) z (0, -0.984808, 0.173648) at (605, 179.6107, 656.295)
component "stock" placed x (1, 0, 0) y (0, 1, 0) z (0, 0, 1) at (0, 0, 0)
component "layout" placed x (1, 0, 0) y (0, 1, 0) z (0, 0, 1) at (0, 0, 0)
component "stand" placed x (1, 0, 0) y (0, 1, 0) z (0, 0, 1) at (0, 0, 0)
component "brick (outdated)" placed x (1, 0, 0) y (0, 1, 0) z (0, 0, 1) at (0, 0, 0)
equation "stockThickness = 46.5 mm"
equation "stockWidth = 7 1/4\""
equation "stockLength = 46\""
equation "d4 = stockWidth"
equation "d5 = stockLength"
equation "boardWidth = 695 mm"
equation "boardDepth = 450 mm"
equation "d14 = boardWidth"
equation "d15 = boardDepth"
equation "boardThickness = 28 mm"
equation "d19 = d4"
equation "d20 = boardThickness"
equation "kerf = 2 mm"
equation "d26 = boardThickness + kerf"
equation "d30 = stockWidth + 23 mm"
equation "d32 = stockThickness"
equation "d34 = stockThickness"
equation "d38 = d36 / 2"
equation "d39 = stockThickness"
equation "d40 = stockWidth"
equation "d41 = d36"
equation "d42 = d14"
equation "d43 = d15"
equation "d46 = 2 * stockThickness"
equation "d47 = -stockWidth"
equation "d56 = stockThickness"
equation "d59 = d57"
equation "d60 = 6\""
equation "d61 = d60"
equation "d62 = d58"
equation "d63 = stockThickness"
equation "d66 = d57"
equation "d67 = 6\""
equation "d68 = d60"
equation "d69 = d58"
equation "d73 = -4 * 2 * stockThickness"
equation "d74 = boardThickness"
equation "footInset = 2\""
equation "footDiameter = 3/4\""
equation "d78 = -footInset"
equation "d79 = footDiameter"
equation "d80 = d79"
equation "d81 = d79"
equation "d82 = d79"
equation "d88 = boardRadius"
equation "d89 = boardBottomChamfer"
equation "d90 = boardTopChamfer"
equation "d93 = d91 / 2 - 0.1 mm"
equation "d98 = 2 * stockThickness"
equation "d99 = -stockWidth"
equation "d100 = boardThickness"
equation "d124 = ( sqrt(2 * boardBottomChamfer * boardBottomChamfer) )"
equation "d126 = boardDepth"
equation "d127 = ( sqrt(2 * boardTopChamfer * boardTopChamfer) )"
equation "d128 = d125"
equation "d129 = standT"
equation "d131 = d130"
equation "d133 = standRadius"
equation "d135 = plyT"
equation "d138 = standRadius"
equation "standRadius = 9 mm"
equation "standWidth = 300 mm"
equation "plyT = 18 mm"
equation "standT = plyT"
equation "d143 = -standWidth / 2"
equation "stretcherOffset = 5 mm"
equation "d167 = plyT"
equation "d172 = stretcherOffset"
equation "d174 = -( plyT - stretcherOffset )"
equation "d176 = -( plyT - stretcherOffset ) / 2"
equation "boardTopChamfer = 2 mm"
equation "boardBottomChamfer = 12 mm"
equation "boardRadius = 30 mm"
